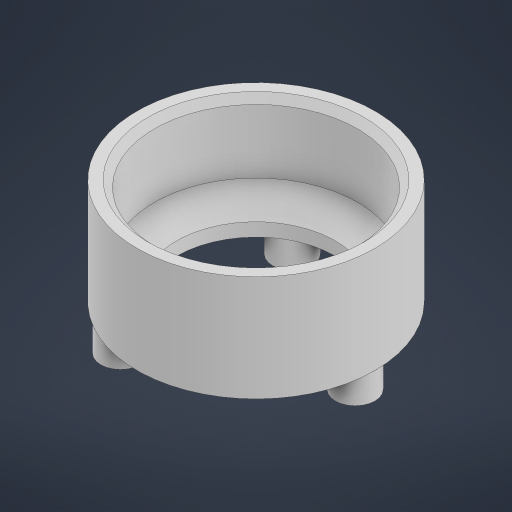
# Autodesk Inventor part: Base
Saved by Autodesk Inventor 2023 (Build 270158000, 158)
## iProperties
Created: 2022-10-27
Part Number: Base
Material: Generic
Document SubType Name: Modeling
Designer: jdbuo
Density: 1 g/cm^3
Appearance: Default
Author: jdbuo
## iProperties of the stored document Base_3DPrint.ipt
Created: 2022-11-10
Part Number: Base_3DPrint
Material: Generic
Document SubType Name: Modeling
Designer: jdbuo
Density: 1 g/cm^3
Appearance: Default
Author: jdbuo
Autodesk Inventor part; units mm, degrees
ref_plane "YZ Plane" through (0, 0, 0) normal (1, 0, 0) x (0, 1, 0)
ref_plane "XZ Plane" through (0, 0, 0) normal (0, 1, 0) x (-1, 0, 0)
ref_plane "XY Plane" through (0, 0, 0) normal (0, 0, 1) x (1, 0, 0)
sketch "Sketch1" plane through (0, 0, 0) normal (0, 0, 1) x (1, 0, 0)
  line L0 (19.05, 0) -> (28.575, 0)
  line L1 (28.575, 0) -> (28.575, 25.4)
  line L2 (28.575, 25.4) -> (24.384, 25.4)
  line L3 (24.384, 25.4) -> (24.384, 8.509)
  line L4 (24.384, 8.509) -> (19.05, 3.175)
  line L5 (19.05, 3.175) -> (19.05, 0)
  line L6 (0, -5.08) -> (0, 30.48) projected
  point P0 (0, 0)
  point P1 (24.384, 16.9545)
  dimension "d0" = 135
  dimension "d1" = 24.384
  dimension "d2" = 28.575
  dimension "d3" = 25.4
  dimension "d4" = 3.175
  dimension "d5" = 19.05
  constraints: 12 end point, 3 perpendicular, 2 horizontal alignment, 1 horizontal, 1 midpoint, 1 parallel
  measures "d0" angle of L5 L4
  measures "d1" horizontal distance of point (24.384, 16.955) point (0, 0)
  measures "d2" distance from line of point (0, 0) L1
  measures "d3" distance of L0.end L1.end
  measures "d4" distance of L4.end L0.start
  measures "d5" distance of point (0, 0) L0.start
revolve "Revolution1" add sketch "Sketch1" angle 360 about axis through (0, -10, 0) along (0, 1, 0)
sketch "Sketch2" plane through (0, 0, 0) normal (0, -1, 0) x (1, 0, 0)
  circle A0 centre (0, 0) radius 28.575 construction
  circle A1 centre (0, 0) radius 19.05 construction
  circle A2 centre (23.8125, 0) radius 4.7625
  constraints: 2 tangent, 1 centre point, 1 horizontal alignment
extrude "Extrusion1" add sketch "Sketch2" along normal blind 6.35
pattern_circular "Circular Pattern1" count 3 over 360 about axis through (0, 12.7, 0) along (0, 1, 0) of "Extrusion1"
chamfer "Chamfer1" distance 1.5875 angle 45 1 edges at (-24.384, 25.4, 0)
body "Solid1"
